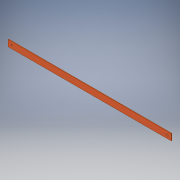
# Autodesk Inventor part: Part1
Saved by Autodesk Inventor 2019 (Build 230136000, 136)
## iProperties
Created: 2021-11-02
Part Number: Part1
Material: Generic
Document SubType Name: Modeling
Designer: modym
Density: 1 g/cm^3
Appearance: Smooth - Light Orange
Author: modym
Autodesk Inventor part; units mm, degrees
ref_plane "YZ Plane" through (0, 0, 0) normal (1, 0, 0) x (0, 1, 0)
ref_plane "XZ Plane" through (0, 0, 0) normal (0, 1, 0) x (-1, 0, 0)
ref_plane "XY Plane" through (0, 0, 0) normal (0, 0, 1) x (1, 0, 0)
sketch "Sketch1" plane through (0, 0, 0) normal (0, 0, 1) x (1, 0, 0)
  line L0 (0, 0) -> (1300, 0)
  line L1 (1300, 0) -> (1300, 50)
  line L2 (1300, 50) -> (0, 50)
  line L3 (0, 50) -> (0, 0)
  line L4 (0, 50) -> (30, 50)
  line L5 (30, 50) -> (30, 25)
  circle A0 centre (30, 25) radius 7.5
  line L6 (650, 50) -> (650, 17.5)
  circle A1 centre (1270, 25) radius 7.5
  dimension "d0" = 1300
  dimension "d1" = 50
  dimension "d4" = 30
  dimension "d5" = 15
  constraints: 14 end point, 2 centre point, 2 parallel, 2 perpendicular, 1 coincident, 1 horizontal, 1 midpoint, 1 point on line, 1 symmetric about line, 1 vertical, 1 other
  measures "d0" distance of L2.end L1.end
  measures "d1" distance of L1.end L0.end
  measures "d4" distance of L2.end L4.end
  measures "d5" diameter of A0
extrude "Extrusion2" add sketch "Sketch1" along normal blind 5
body "Solid2"
